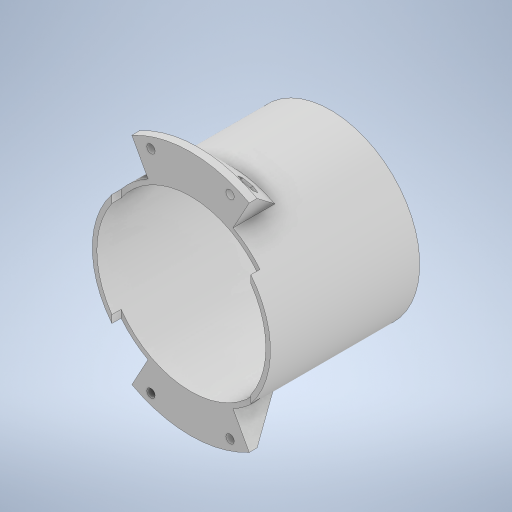
# Autodesk Inventor part: LensMount_JJC_FDA_LED1
Saved by Autodesk Inventor 2023 (Build 270158000, 158)
## iProperties
Created: 2022-10-30
Part Number: LensMount_JJC_FDA_LED1
Material: Generic
Document SubType Name: Modeling
Designer: Piotr
Density: 1 g/cm^3
Appearance: Default
Author: Piotr
Autodesk Inventor part; units mm, degrees
ref_plane "YZ Plane" through (0, 0, 0) normal (1, 0, 0) x (0, 1, 0)
ref_plane "XZ Plane" through (0, 0, 0) normal (0, 1, 0) x (-1, 0, 0)
sketch "Sketch1" plane through (0, 0, 0) normal (0, 0, 1) x (1, 0, 0)
  circle A0 centre (0, 0) radius 32.25
  circle A1 centre (0, 0) radius 34
  line L0 (0, 0) -> (34, 0) construction
  line L1 (0, 0) -> (30.0202, 15.962) construction
  circle A2 centre (0, 0) radius 30.7
  line L2 (0, 0) -> (26.7199, 15.1174) construction
  line L3 (0, 0) -> (27.4745, 13.6983) construction
  line L4 (28.069, 15.8807) -> (29.5921, 16.7424) construction
  line L5 (28.8616, 14.3899) -> (30.4278, 15.1707) construction
  line L6 (27.4745, 13.6983) -> (28.8616, 14.3899)
  line L7 (26.7199, 15.1174) -> (28.069, 15.8807)
  line L8 (-26.7199, -15.1174) -> (-28.069, -15.8807)
  line L9 (-27.4745, -13.6983) -> (-28.8616, -14.3899)
  point P0 (-28.069, -15.8807)
  point P1 (-27.4745, -13.6983)
  dimension "d0" = 64.5
  dimension "d1" = 68
  dimension "d2" = 28
  dimension "d3" = 61.4
  dimension "d4" = 3
  dimension "d11" = 360
  constraints: 20 end point, 7 point on circle, 4 collinear, 3 centre point, 3 coincident, 1 horizontal, 1 symmetric about line, 13 other
  measures "d0" diameter of A0
  measures "d1" diameter of A1
  measures "d2" angle of L0 L1
  measures "d3" diameter of A2
  measures "d4" angle of L3 L2
extrude "Extrusion1" add sketch "Sketch1" along normal blind 1.5 contours L6 A2 L7 A0 | A0 L9 A2 L8 | A1
sketch "Sketch2" plane through (0, 0, 0) normal (0, 0, -1) x (-1, 0, 0)
  line L0 (-27.4745, 13.6983) -> (-28.8616, 14.3899) projected
  arc A0 (-28.8616, 14.3899) -> (28.069, -15.8807) centre (0, 0) ccw projected
  line L1 (28.069, -15.8807) -> (26.7199, -15.1174) projected
  arc A1 (26.7199, -15.1174) -> (27.4745, -13.6983) centre (0, 0) ccw projected
  line L2 (27.4745, -13.6983) -> (28.8616, -14.3899) projected
  arc A2 (28.8616, -14.3899) -> (-28.069, 15.8807) centre (0, 0) ccw projected
  line L3 (-28.069, 15.8807) -> (-26.7199, 15.1174) projected
  arc A3 (-26.7199, 15.1174) -> (-27.4745, 13.6983) centre (0, 0) ccw projected
  circle A4 centre (0, 0) radius 34 projected
  line L4 (0, 0) -> (-34, 0) construction
  arc A5 (-30.7, 0) -> (-29.8518, -7.1668) centre (0, 0) ccw
  arc A6 (-28.9137, -12.8732) -> (-30.0144, -10.0427) centre (0, 0) ccw construction
  line L5 (0, 0) -> (-28.0458, -12.4868) construction
  line L6 (-28.0458, -12.4868) -> (-28.5026, -12.6902) construction
  line L7 (0, 0) -> (-30.0144, -10.0427) construction
  line L8 (0, 0) -> (-30.7755, -7.3885) construction
  line L9 (-30.0144, -10.0427) -> (-29.8518, -7.1668)
  arc A7 (-23.1861, -20.8769) -> (-28.5026, -12.6902) centre (0, 0) ccw construction
  line L10 (0, 0) -> (-23.9664, -21.5795) construction
  line L11 (-28.5026, -12.6902) -> (-28.9137, -12.8732)
  line L12 (0, 0) -> (-19.8551, -25.4133) construction
  line L13 (-23.1861, -20.8769) -> (-19.8551, -25.4133)
  arc A8 (-30.0144, -10.0427) -> (-28.9137, -12.8732) centre (0, 0) ccw
  arc A9 (-28.5026, -12.6902) -> (-23.1861, -20.8769) centre (0, 0) ccw
  arc A10 (-27.4745, 13.6983) -> (-30.7, 0) centre (0, 0) ccw
  arc A11 (-29.8518, -7.1668) -> (-26.7199, 15.1174) centre (0, 0) ccw construction
  arc A12 (-26.7199, 15.1174) -> (-27.4745, 13.6983) centre (0, 0) ccw
  arc A13 (26.7199, -15.1174) -> (27.4745, -13.6983) centre (0, 0) ccw
  arc A14 (27.4745, -13.6983) -> (30.7, 0) centre (0, 0) ccw
  arc A15 (30.7, 0) -> (29.8518, 7.1668) centre (0, 0) ccw
  line L14 (30.0144, 10.0427) -> (29.8518, 7.1668)
  arc A16 (30.0144, 10.0427) -> (28.9137, 12.8732) centre (0, 0) ccw
  line L15 (28.5026, 12.6902) -> (28.9137, 12.8732)
  arc A17 (28.5026, 12.6902) -> (23.1861, 20.8769) centre (0, 0) ccw
  line L16 (23.1861, 20.8769) -> (19.8551, 25.4133)
  line L17 (0, 0) -> (6.3829, -30.0291) construction
  arc A18 (-28.8616, 14.3899) -> (28.069, -15.8807) centre (0, 0) ccw projected
  arc A19 (6.3829, -30.0291) -> (26.7199, -15.1174) centre (0, 0) ccw
  line L18 (6.3829, -30.0291) -> (6.7052, -31.5453)
  line L19 (0, 0) -> (-6.3829, 30.0291) construction
  line L20 (-6.3829, 30.0291) -> (-6.7052, 31.5453)
  arc A20 (-6.3829, 30.0291) -> (-26.7199, 15.1174) centre (0, 0) ccw
  point P0 (28.0458, 12.4868)
  point P1 (27.4745, -13.6983)
  point P2 (-26.7199, 15.1174)
  dimension "d15" = 63.3
  dimension "d16" = 24
  dimension "d17" = 18.5
  dimension "d18" = 13.5
  dimension "d19" = 62.4
  dimension "d20" = 42
  dimension "d21" = 52
  dimension "d24" = 360
  dimension "d43" = 50
  dimension "d46" = 360
  constraints: 39 point on circle, 36 end point, 15 centre point, 6 coincident, 3 collinear, 3 concentric, 3 point on line, 1 horizontal, 1 horizontal alignment, 61 other
  measures "d15" diameter of A6
  measures "d16" angle of L5 L4
  measures "d17" angle of L7 L4
  measures "d18" angle of L8 L4
  measures "d19" diameter of A7
  measures "d20" angle of L4 L10
  measures "d21" angle of L4 L12
  measures "d43" angle of L12 L17
extrude "Extrusion2" add sketch "Sketch2" along normal blind 1.65 contours A10 A5 L9 A8 L11 A9 L13 A0 L0 | L3 A2 L20 A20 | L18 A19 L1 A0 | A2 L2 A14 A15 L14 A16 L15 A17 L16 | A4
sketch "Sketch4" plane through (0, 0, 1.5) normal (0, 0, 1) x (1, 0, 0)
  circle A0 centre (0, 0) radius 34 projected
  arc A1 (28.069, 15.8807) -> (-28.8616, -14.3899) centre (0, 0) ccw projected
  circle A2 centre (0, 0) radius 32.25
  point P0 (-28.8616, -14.3899)
  constraints: 1 centre point, 1 coincident, 1 concentric
extrude "Extrusion4" add sketch "Sketch4" along normal blind 50.3
sketch "Sketch11" plane through (0, 0, 51.8) normal (0, 0, 1) x (1, 0, 0)
  circle A0 centre (0, 0) radius 34 projected
  circle A1 centre (-15.1, 40.3683) radius 1.6
  circle A2 centre (15.1, -40.3683) radius 1.6
  circle A3 centre (0, 0) radius 43.1 construction
  line L0 (0, 0) -> (0, 34) construction
  circle A4 centre (15.1, 40.3683) radius 1.6
  circle A5 centre (-15.1, -40.3683) radius 1.6
  circle A6 centre (0, 0) radius 46.9
  line L1 (0, 0) -> (-15.1, 40.3683) construction
  line L2 (-22.3849, 41.2132) -> (22.3849, -41.2132)
  line L3 (22.3849, 41.2132) -> (-22.3849, -41.2132)
  point P0 (-16.2279, -29.8773)
  point P1 (16.2279, -29.8773)
  point P2 (16.2279, 29.8773)
  point P3 (-16.2279, 29.8773)
  dimension "d76" = 86.2
  dimension "d74" = 360
  dimension "d77" = 30.2
  dimension "d78" = 3.2
  dimension "d79" = 93.8
  dimension "d81" = 8
  constraints: 8 end point, 5 centre point, 4 symmetric about line, 2 coincident, 2 point on circle, 1 midpoint, 1 vertical, 12 other
  measures "d77" distance of A4.centre L1.end
  measures "d78" diameter of A1
  measures "d79" diameter of A6
  measures "d81" angle of L1 L2
extrude "Extrusion12" add sketch "Sketch11" against normal blind 3 contours A0 L2 A6 L3 | L2 A6 L3 A0 | A1 | A2 | A4 | A5 picked at (-7.1791, 40.2894) picked at (7.1791, -40.2894)
chamfer "Chamfer2" distance 12.9 angle 45 2 edges at (0, -34, 48.8) (0, 34, 48.8)
extrude "Extrusion13" cut sketch "Sketch11" against normal through all contours A1 | A2 | A4 | A5
ref_plane "Work Plane2" through (0, 0, 48.8) normal (0, 0, 1) x (1, 0, 0)
sketch "Sketch12" plane through (0, 0, 48.8) normal (0, 0, 1) x (1, 0, 0)
  circle A0 centre (-15.1, 40.3683) radius 1.6 projected
  circle A1 centre (15.1, -40.3683) radius 1.6 projected
  circle A2 centre (15.1, 40.3683) radius 1.6 projected
  circle A3 centre (-15.1, -40.3683) radius 1.6 projected
  arc A4 (22.3849, 41.2132) -> (-22.3849, 41.2132) centre (0, 0) ccw projected
  line L0 (22.3849, 41.2132) -> (16.2279, 29.8773) projected
  arc A5 (16.2279, -29.8773) -> (16.2279, 29.8773) centre (0, 0) ccw projected
  line L1 (16.2279, -29.8773) -> (22.3849, -41.2132) projected
  arc A6 (-22.3849, -41.2132) -> (22.3849, -41.2132) centre (0, 0) ccw projected
  line L2 (-22.3849, -41.2132) -> (-16.2279, -29.8773) projected
  arc A7 (-16.2279, 29.8773) -> (-16.2279, -29.8773) centre (0, 0) ccw projected
  line L3 (-16.2279, 29.8773) -> (-22.3849, 41.2132) projected
  circle A8 centre (0, 0) radius 32.25 projected
  line L4 (13.7184, -37.318) -> (17.0509, -37.6467)
  line L5 (17.0509, -37.6467) -> (18.4325, -40.697)
  line L6 (18.4325, -40.697) -> (16.4816, -43.4187)
  line L7 (16.4816, -43.4187) -> (13.1491, -43.0899)
  line L8 (13.1491, -43.0899) -> (11.7675, -40.0396)
  line L9 (11.7675, -40.0396) -> (13.7184, -37.318)
  line L10 (0, 0) -> (18.4325, -40.697) construction
  line L11 (0, 0) -> (0, -32.25) construction
  arc A9 (-6.7052, -31.5453) -> (19.8551, -25.4133) centre (0, 0) ccw construction
  line L12 (0, 0) -> (-32.25, 0) construction
  arc A10 (-19.8551, 25.4133) -> (-28.8616, -14.3899) centre (0, 0) ccw construction
  line L13 (-13.7184, -37.318) -> (-17.0509, -37.6467)
  line L14 (-17.0509, -37.6467) -> (-18.4325, -40.697)
  line L15 (-18.4325, -40.697) -> (-16.4816, -43.4187)
  line L16 (-16.4816, -43.4187) -> (-13.1491, -43.0899)
  line L17 (-13.1491, -43.0899) -> (-11.7675, -40.0396)
  line L18 (-11.7675, -40.0396) -> (-13.7184, -37.318)
  line L19 (13.7184, 37.318) -> (17.0509, 37.6467)
  line L20 (17.0509, 37.6467) -> (18.4325, 40.697)
  line L21 (18.4325, 40.697) -> (16.4816, 43.4187)
  line L22 (16.4816, 43.4187) -> (13.1491, 43.0899)
  line L23 (13.1491, 43.0899) -> (11.7675, 40.0396)
  line L24 (11.7675, 40.0396) -> (13.7184, 37.318)
  line L25 (-13.7184, 37.318) -> (-17.0509, 37.6467)
  line L26 (-11.7675, 40.0396) -> (-13.7184, 37.318)
  line L27 (-13.1491, 43.0899) -> (-11.7675, 40.0396)
  line L28 (-16.4816, 43.4187) -> (-13.1491, 43.0899)
  line L29 (-18.4325, 40.697) -> (-16.4816, 43.4187)
  line L30 (-17.0509, 37.6467) -> (-18.4325, 40.697)
  dimension "d90" = 5.8
  constraints: 54 end point, 18 symmetric about line, 2 point on circle, 1 coincident, 1 collinear, 1 perpendicular, 1 vertical, 13 other
  measures "d90" distance between parallel lines of L9 L6
extrude "Extrusion14" cut sketch "Sketch12" against normal blind 10 contours A0 | A1 | A2 | A3 | L4 L5 L6 L7 L8 L9 | L18 L17 L16 L15 L14 L13 | L24 L23 L22 L21 L20 L19 | L25 L30 L29 L28 L27 L26
sketch "Sketch13" plane through (0, 0, 51.8) normal (0, 0, 1) x (1, 0, 0)
  circle A0 centre (0, 0) radius 32.25 projected
  arc A1 (-16.2279, 29.8773) -> (-16.2279, -29.8773) centre (0, 0) ccw projected
  arc A2 (16.2279, 29.8773) -> (-16.2279, 29.8773) centre (0, 0) ccw projected
  arc A3 (16.2279, -29.8773) -> (16.2279, 29.8773) centre (0, 0) ccw projected
  arc A4 (-16.2279, -29.8773) -> (16.2279, -29.8773) centre (0, 0) ccw projected
  circle A5 centre (0, 0) radius 34 projected
  line L0 (-18, 12.15) -> (18, 12.15) construction
  line L1 (18, 12.15) -> (18, -12.15) construction
  line L2 (18, -12.15) -> (-18, -12.15) construction
  line L3 (-18, -12.15) -> (-18, 12.15) construction
  line L4 (-18, 12.15) -> (18, -12.15) construction
  line L5 (18, 12.15) -> (-18, -12.15) construction
  line L6 (-26.5, 17.4) -> (26.5, 17.4) construction
  line L7 (26.5, 17.4) -> (26.5, -17.4) construction
  line L8 (26.5, -17.4) -> (-26.5, -17.4) construction
  line L9 (-26.5, -17.4) -> (-26.5, 17.4) construction
  line L10 (-26.5, 17.4) -> (26.5, -17.4) construction
  line L11 (26.5, 17.4) -> (-26.5, -17.4) construction
  line L12 (-26.5, 17.4) -> (-26.5, 26.4)
  line L13 (0, 0) -> (0, 17.4) construction
  line L14 (0, 0) -> (26.5, 0) construction
  line L15 (26.5, 17.4) -> (26.5, 26.4)
  line L16 (-26.5, -17.4) -> (-26.5, -26.4)
  line L17 (26.5, -17.4) -> (26.5, -26.4)
  point P0 (26.5, -18.3797)
  point P1 (26.5, -21.3014)
  point P2 (26.5, 21.3014)
  point P3 (26.5, 18.3797)
  point P4 (-26.5, -21.3014)
  point P5 (-26.5, -18.3797)
  point P6 (-26.5, 18.3797)
  point P7 (-26.5, 21.3014)
  dimension "d93" = 36
  dimension "d94" = 24.3
  dimension "d95" = 53
  dimension "d96" = 34.8
  dimension "d97" = 9
  constraints: 36 end point, 6 midpoint, 4 parallel, 3 symmetric about line, 2 horizontal, 2 perpendicular, 1 point on line
  measures "d93" distance of L1.end L2.end
  measures "d94" distance of L0.end L1.end
  measures "d95" distance of L7.end L8.end
  measures "d96" distance of L6.end L7.end
  measures "d97" distance of L6.start L12.end
extrude "Extrusion15" add sketch "Sketch13" along normal blind 3.5 contours A0 L15 A3 L17 | A0 L16 A1 L12
sketch "Sketch14" plane through (0, 0, 48.8) normal (0, 0, -1) x (-1, 0, 0)
  circle A0 centre (15.1, -40.3683) radius 1.6 projected
  circle A1 centre (-15.1, -40.3683) radius 1.6 projected
  circle A2 centre (15.1, 40.3683) radius 1.6 projected
  circle A3 centre (-15.1, 40.3683) radius 1.6 projected
  point P0 (0, 0)
extrude "Extrusion16" add sketch "Sketch14" against normal blind 0.2
body "Solid1"
